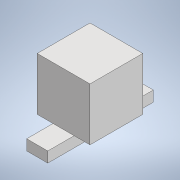
# Autodesk Inventor part: Part4
Saved by Autodesk Inventor 2022 (Build 260153000, 153)
## iProperties
Created: 2021-07-07
Part Number: Part4
Material: Generic
Document SubType Name: Modeling
Designer: Bhagiratha
Density: 1 g/cm^3
Appearance: Default
Author: Bhagiratha
Autodesk Inventor part; units mm, degrees
ref_plane "YZ Plane" through (0, 0, 0) normal (1, 0, 0) x (0, 1, 0)
ref_plane "XZ Plane" through (0, 0, 0) normal (0, 1, 0) x (-1, 0, 0)
ref_plane "XY Plane" through (0, 0, 0) normal (0, 0, 1) x (1, 0, 0)
sketch "Sketch1" plane through (0, 0, 0) normal (0, 1, 0) x (-1, 0, 0)
  line L0 (-10, -50) -> (10, -50)
  line L1 (10, -50) -> (10, 50)
  line L2 (10, 50) -> (-10, 50)
  line L3 (-10, 50) -> (-10, -50)
  line L4 (-10, -50) -> (10, 50) construction
  line L5 (10, -50) -> (-10, 50) construction
  point P0 (0, 0)
  dimension "d0" = 20
  dimension "d1" = 100
  constraints: 12 end point, 2 midpoint, 2 parallel, 1 horizontal, 1 perpendicular
  measures "d0" distance of L2.end L1.end
  measures "d1" distance of L0.end L1.end
extrude "Extrusion1" add sketch "Sketch1" along normal blind 10
sketch "Sketch2" plane through (0, 10, 0) normal (0, 1, 0) x (1, 0, 0)
  line L0 (25, 25) -> (-25, 25)
  line L1 (-25, 25) -> (-25, -25)
  line L2 (-25, -25) -> (25, -25)
  line L3 (25, -25) -> (25, 25)
  line L4 (25, 25) -> (-25, -25) construction
  line L5 (-25, 25) -> (25, -25) construction
  point P0 (0, 0)
  dimension "d4" = 50
  dimension "d5" = 50
  constraints: 12 end point, 2 midpoint, 2 parallel, 1 horizontal, 1 perpendicular
  measures "d4" distance of L2.end L1.end
  measures "d5" distance of L1.end L0.end
extrude "Extrusion2" add sketch "Sketch2" along normal blind 30
sketch "Sketch3" plane through (-25, 10, -25) normal (-1, 0, 0) x (0, 0, 1)
  circle A0 centre (25, 15.6421) radius 10
  point P0 (25, -10)
  dimension "d8" = 20
  constraints: 1 centre point
  measures "d8" diameter of A0
extrude "Extrusion3" cut sketch "Sketch3" against normal through all
body "Solid1"
